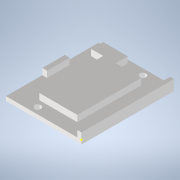
# Autodesk Inventor part: USB-Hub
Saved by Autodesk Inventor 2022 (Build 260153000, 153)
## iProperties
Created: 2021-11-08
Part Number: USB-Hub
Material: Generisch
Document SubType Name: Modeling
Designer: lukas
Density: 1 g/cm^3
Appearance: Vorgabe
Author: lukas
Autodesk Inventor part; units mm, degrees
ref_plane "YZ Plane" through (0, 0, 0) normal (1, 0, 0) x (0, 1, 0)
ref_plane "XZ Plane" through (0, 0, 0) normal (0, 1, 0) x (-1, 0, 0)
ref_plane "XY Plane" through (0, 0, 0) normal (0, 0, 1) x (1, 0, 0)
sketch "Skizze1" plane through (0, 0, 0) normal (0, 1, 0) x (-1, 0, 0)
  line L0 (0, 0) -> (18, 0)
  line L1 (18, 0) -> (18, -22.1)
  line L2 (18, -22.1) -> (0, -22.1)
  line L3 (0, -22.1) -> (0, 0)
  circle A0 centre (12, -1.5) radius 0.8
  circle A1 centre (6, -20.6) radius 0.8
  dimension "d0" = 18
  dimension "d1" = 22.1
  dimension "d4" = 6
  dimension "d6" = 1.6
  dimension "d7" = 1.5
  dimension "d8" = 1.6
  dimension "d9" = 1.5
  dimension "d10" = 6
  constraints: 8 end point, 2 centre point, 2 parallel, 1 horizontal, 1 perpendicular
  measures "d0" distance of L1.end L2.end
  measures "d1" distance of L0.end L1.end
  measures "d4" distance from line of A1.centre L3
  measures "d6" diameter of A1
  measures "d7" distance from line of A1.centre L2
  measures "d8" diameter of A0
  measures "d9" distance from line of L0 A0.centre
  measures "d10" distance from line of A0.centre L1
extrude "Extrusion1" add sketch "Skizze1" along normal blind 1
sketch "Skizze2" plane through (0, 1, 0) normal (0, 1, 0) x (1, 0, 0)
  point P0 (0, 0)
sketch "Skizze3" plane through (0, 1, 0) normal (0, 1, 0) x (1, 0, 0)
  line L0 (-13.2189, 3.1467) -> (-4.1223, 3.1467)
  line L1 (-4.1223, 3.1467) -> (-4.1223, 18.4267)
  line L2 (-4.1223, 18.4267) -> (-13.2189, 18.4267)
  line L3 (-13.2189, 18.4267) -> (-13.2189, 3.1467)
  line L4 (-16.1045, 18.4267) -> (-10.2233, 18.4267)
  line L5 (-10.2233, 18.4267) -> (-10.2233, 21.2849)
  line L6 (-10.2233, 21.2849) -> (-16.1045, 21.2849)
  line L7 (-16.1045, 21.2849) -> (-16.1045, 18.4267)
  line L8 (-18, 0) -> (0, 0) projected
  line L9 (0, 0) -> (0, 22.1) projected
  line L10 (-0.9344, 0) -> (0, 0)
  line L11 (0, 0) -> (0, 22.1)
  line L12 (0, 22.1) -> (-0.9344, 22.1)
  line L13 (-0.9344, 22.1) -> (-0.9344, 0)
  line L14 (-18, 22.1) -> (-18, 0) projected
  line L15 (-18, 8.6706) -> (-16.8465, 8.6706)
  line L16 (-16.8465, 8.6706) -> (-16.8465, 14.0571)
  line L17 (-16.8465, 14.0571) -> (-18, 14.0571)
  line L18 (-18, 14.0571) -> (-18, 8.6706)
  point P0 (-16.8465, 11.3638)
  point P1 (-18, 11.3638)
  constraints: 32 end point, 8 parallel, 4 horizontal, 4 perpendicular, 3 point on line, 2 midpoint, 1 horizontal alignment
extrude "Extrusion2" add sketch "Skizze3" along normal blind 1.5
ref_plane "Arbeitsebene1" through (0, 0, -11.05) normal (0, 0, -1) x (-1, 0, 0)
equation "\"d8\" = d6"
equation "\"d9\" = d7"
equation "\"d10\" = d4"
